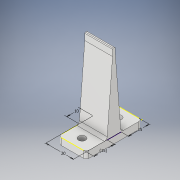
# Autodesk Inventor part: Endtstop_Z
Saved by Autodesk Inventor 2019 (Build 230136000, 136)
## iProperties
Created: 2018-05-10
Part Number: Endtstop_Z
Material: Polyaryletherketon-Kunststoff
Document SubType Name: Modeling
Designer: marc
Density: 1.32 g/cm^3
Appearance: Glatt - Weiß
Mass: 13.2064 g
Surface Area: 48.8647 cm^2
Volume: 10.0048 cm^3
Author: marc
## iProperties of the stored document Endtstop_Z_3D-Druck.ipt
Created: 2018-05-10
Part Number: Endtstop_Z_3D-Druck
Material: Generisch
Document SubType Name: Modeling
Designer: marc
Density: 1 g/cm^3
Appearance: Vorgabe
Author: marc
Autodesk Inventor part; units mm, degrees
ref_plane "YZ Plane" through (0, 0, 0) normal (1, 0, 0) x (0, 1, 0)
ref_plane "XZ Plane" through (0, 0, 0) normal (0, 1, 0) x (-1, 0, 0)
ref_plane "XY Plane" through (0, 0, 0) normal (0, 0, 1) x (1, 0, 0)
sketch "Skizze1" plane through (0, 0, 0) normal (0, 1, 0) x (-1, 0, 0)
  line L0 (0, 0) -> (20, 0)
  line L1 (20, 0) -> (20, 40)
  line L2 (20, 40) -> (0, 40)
  line L3 (0, 40) -> (0, 0)
  circle A0 centre (10, 33) radius 2.55
  circle A1 centre (10, 7) radius 2.55
  dimension "d0" = 20
  dimension "d1" = 40
  dimension "d2" = 5.1
  dimension "d3" = 5.1
  dimension "d4" = 7
  dimension "d5" = 7
  dimension "d6" = 10
  dimension "d7" = 10
  constraints: 8 end point, 2 centre point, 2 parallel, 1 horizontal, 1 perpendicular
  measures "d0" distance of L2.end L1.end
  measures "d1" distance of L0.end L1.end
  measures "d2" diameter of A1
  measures "d3" diameter of A0
  measures "d4" distance from line of L2 A0.centre
  measures "d5" distance from line of L0 A1.centre
  measures "d6" distance from line of L3 A0.centre
  measures "d7" distance from line of L3 A1.centre
extrude "Extrusion1" add sketch "Skizze1" along normal blind 5
fillet "Rundung1" radius 2 4 edges at (-20, 2.5, 40) (-20, 2.5, 0) (0, 2.5, 0) (0, 2.5, 40)
sketch "Skizze2" plane through (0, 5, 0) normal (0, 1, 0) x (1, 0, 0)
  line L0 (-20, -2) -> (-20, -38) projected
  line L1 (-20, -25) -> (0, -25)
  line L2 (0, -25) -> (0, -15)
  line L3 (0, -15) -> (-20, -15)
  line L4 (-20, -15) -> (-20, -25)
  line L5 (-2, 0) -> (-18, 0) projected
  line L6 (-18, -40) -> (-2, -40) projected
  point P0 (0, 0)
  dimension "d11" = 10
  dimension "d12" = 20
  dimension "d13" = 15
  dimension "d14" = 15
  constraints: 8 end point, 2 parallel, 1 horizontal, 1 perpendicular, 1 point on line
  measures "d11" distance of L3.end L1.start
  measures "d12" distance of L2.end L3.end
  measures "d13" distance between parallel lines of L5 L3
  measures "d14" distance between parallel lines of L6 L1
sketch "Skizze5" plane through (0, 0, 0) normal (1, 0, 0) x (0, 1, 0)
  line L0 (55, 21) -> (55, 19)
  line L1 (5, 0) -> (0, 0) projected
  line L2 (5, 2) -> (5, 38) projected
  line L3 (5, 25) -> (55, 21)
  line L4 (5, 15) -> (55, 19)
  point P0 (5, 15)
  dimension "d25" = 19
  dimension "d26" = 2
  dimension "d27" = 50
  constraints: 6 end point, 1 equal length, 1 parallel, 1 point on line, 1 vertical
  measures "d25" distance from line of L1 L0.end
  measures "d26" distance of L0.start L0.end
  measures "d27" distance between parallel lines of L0 L2
extrude "Extrusion3" add sketch "Skizze5" against normal up to surface (20 mm away)
sketch "Skizze6" plane through (0, 55, 21) normal (0, 1, 0) x (1, 0, 0)
  line L0 (-20, 2) -> (0, 2) projected
  line L1 (0, 2) -> (0, 0) projected
  line L2 (0, 0) -> (-20, 0) projected
  line L3 (-20, 0) -> (-20, 2) projected
  point P0 (0, 21)
extrude "Extrusion4" add sketch "Skizze6" along normal blind 5
fillet "Rundung2" radius 2 2 edges at (-10, 5, 15) (-10, 5, 25)
fillet "Rundung3" radius 0.5 2 edges at (-10, 60, 21) (-10, 60, 19)
equation "\"d3\" = d2"
equation "\"d5\" = d4"
equation "\"d6\" = d7"
